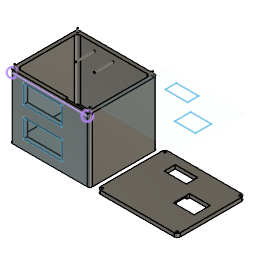
Project housingV4 (Autodesk Fusion 360 design; units mm, degrees)
Autodesk Fusion 360 part; units mm, degrees
sketch "Sketch1" plane through (0, 0, 0) normal (0, 0, 1) x (1, 0, 0)
  line L0 (2, 0) -> (63, 0)
  line L1 (65, 2) -> (65, 53)
  line L2 (63, 55) -> (2, 55)
  line L3 (0, 53) -> (0, 2)
  arc A0 (2, 55) -> (0, 53) centre (2, 53) ccw
  arc A1 (63, 0) -> (65, 2) centre (63, 2) ccw
  arc A2 (65, 53) -> (63, 55) centre (63, 53) ccw
  arc A3 (0, 2) -> (2, 0) centre (2, 2) ccw
  point P0 (65, 0)
  point P1 (0, 55)
  dimension "d1" = 55
  dimension "d2" = 65
  dimension "d3" = 2
  constraint horizontal L0
  constraint vertical L1
  constraint horizontal L2
  constraint vertical L3
  constraint coincident P1 L2
  constraint coincident P1 L3
  constraint tangent L2 A0
  constraint tangent L3 A0
  constraint coincident P0 L0
  constraint coincident P0 L1
  constraint tangent L0 A1
  constraint tangent L1 A1
  constraint equal A0 A1
  constraint tangent L1 A2
  constraint tangent L2 A2
  constraint equal A0 A2
  constraint coincident origin L0
  constraint coincident origin L3
  constraint tangent L0 A3
  constraint tangent L3 A3
  constraint equal A0 A3
  measures "d1" distance of origin P1
  measures "d2" distance of origin P0
  measures "d3" radius of A0
extrude "Extrude1" add sketch "Sketch1" along normal blind 50 makes body 1
sketch "Sketch2" plane through (0, 0, 50) normal (0, 0, 1) x (-1, 0, 0)
  arc A0 (0, -2) -> (-2, 0) centre (-2, -2) ccw
  line L0 (-2, 0) -> (-63, 0)
  arc A1 (-63, 0) -> (-65, -2) centre (-63, -2) ccw
  line L1 (-65, -2) -> (-65, -53)
  arc A2 (-65, -53) -> (-63, -55) centre (-63, -53) ccw
  line L2 (-63, -55) -> (-2, -55)
  arc A3 (-2, -55) -> (0, -53) centre (-2, -53) ccw
  line L3 (0, -53) -> (0, -2)
  line L4 (-3, -49.5) -> (-3, -5.5)
  line L5 (-5.5, -3) -> (-59.5, -3)
  line L6 (-62, -5.5) -> (-62, -49.5)
  line L7 (-59.5, -52) -> (-5.5, -52)
  arc A4 (-5.5, -52) -> (-3, -49.5) centre (-5.5, -49.5) ccw
  arc A5 (-3, -5.5) -> (-5.5, -3) centre (-5.5, -5.5) ccw
  arc A6 (-59.5, -3) -> (-62, -5.5) centre (-59.5, -5.5) ccw
  arc A7 (-62, -49.5) -> (-59.5, -52) centre (-59.5, -49.5) ccw
  dimension "d7" = 2.5
  constraint tangent L4 A4
  constraint tangent L7 A4
  constraint tangent L4 A5
  constraint tangent L5 A5
  constraint equal A4 A5
  constraint tangent L5 A6
  constraint tangent L6 A6
  constraint equal A4 A6
  constraint tangent L6 A7
  constraint tangent L7 A7
  constraint equal A4 A7
  measures "d7" radius of A4
extrude "Extrude2" cut sketch "Sketch2" against normal blind 47 contours L4 L5 L6 L7 A4 A5 A6 A7 bodies 1
sketch "Sketch3" plane through (0, 0, 0) normal (0, -1, 0) x (1, 0, 0)
  line L0 (2, 0) -> (63, 0)
  line L1 (63, 0) -> (63, 50)
  line L2 (63, 50) -> (2, 50)
  line L3 (2, 50) -> (2, 0)
sketch "Sketch4" plane through (0, 0, 0) normal (0, -1, 0) x (1, 0, 0)
  line L0 (11.3476, 47.3) -> (42.3476, 47.3)
  line L1 (42.3476, 47.3) -> (42.3476, 32.3)
  line L2 (42.3476, 32.3) -> (11.3476, 32.3)
  line L3 (11.3476, 32.3) -> (11.3476, 47.3)
  line L4 (11.3476, 23.1) -> (42.3476, 23.1)
  line L5 (11.3476, 8.1) -> (11.3476, 23.1)
  line L6 (42.3476, 8.1) -> (11.3476, 8.1)
  line L7 (42.3476, 23.1) -> (42.3476, 8.1)
  line L8 (63, 50) -> (2, 50)
  dimension "d10" = 31
  dimension "d11" = 15
  dimension "d12" = 31
  dimension "d13" = 15
  dimension "d14" = 9.2
  constraint horizontal L0
  constraint vertical L1
  constraint horizontal L2
  constraint vertical L3
  constraint horizontal L4
  constraint vertical L7
  constraint horizontal L6
  constraint vertical L5
  constraint vertical L2.end L4.start
  measures "d10" distance of L0.start L0.end
  measures "d11" distance of L0.end L1.end
  measures "d12" distance of L4.end L4.start
  measures "d13" distance of L4.end L6.start
  measures "d14" distance of L2 L4
extrude "Extrude3" cut sketch "Sketch4" against normal blind 6 bodies 1
sketch "Sketch5" plane through (0, 52, 0) normal (0, -1, 0) x (1, 0, 0)
  line L0 (59.5, 50) -> (5.5, 50)
  line L1 (5.5, 50) -> (5.5, 3)
  line L2 (5.5, 3) -> (59.5, 3)
  line L3 (59.5, 3) -> (59.5, 50)
  line L4 (15, 48) -> (33.5, 48)
  line L5 (33.5, 48) -> (33.5, 4)
  line L6 (33.5, 4) -> (15, 4)
  line L7 (15, 4) -> (15, 48)
  circle A0 centre (16.689, 46.5) radius 0.7
  circle A1 centre (31.811, 46.5) radius 0.7
  circle A2 centre (16.689, 5.5) radius 0.7
  circle A3 centre (31.811, 5.5) radius 0.7
  dimension "d18" = 44
  dimension "d19" = 18.5
  dimension "d20" = 1.4
  constraint horizontal L4
  constraint vertical L5
  constraint horizontal L6
  constraint vertical L7
  measures "d18" distance of L4.end L5.end
  measures "d19" distance of L4.start L4.end
  measures "d20" diameter of A0
extrude "Extrude4" add sketch "Sketch5" along normal blind 12 contours A0 | A1 | A2 | A3 bodies 1
sketch "Sketch6" plane through (0, 0, 50) normal (0, 0, 1) x (-1, 0, 0)
  line L0 (-5.5, -52) -> (-59.5, -52)
  arc A0 (-62, -49.5) -> (-59.5, -52) centre (-59.5, -49.5) ccw
  line L1 (-62, -49.5) -> (-62, -5.5)
  arc A1 (-59.5, -3) -> (-62, -5.5) centre (-59.5, -5.5) ccw
  line L2 (-59.5, -3) -> (-5.5, -3)
  arc A2 (-3, -5.5) -> (-5.5, -3) centre (-5.5, -5.5) ccw
  line L3 (-3, -5.5) -> (-3, -49.5)
  arc A3 (-5.5, -52) -> (-3, -49.5) centre (-5.5, -49.5) ccw
  arc A4 (0, -2) -> (-2, 0) centre (-2, -2) ccw
  line L4 (-2, 0) -> (-63, 0)
  arc A5 (-63, 0) -> (-65, -2) centre (-63, -2) ccw
  line L5 (-65, -2) -> (-65, -53)
  arc A6 (-65, -53) -> (-63, -55) centre (-63, -53) ccw
  line L6 (-63, -55) -> (-2, -55)
  arc A7 (-2, -55) -> (0, -53) centre (-2, -53) ccw
  line L7 (0, -53) -> (0, -2)
  line L8 (-2.5, -55) -> (-62.5, -55)
  line L9 (-65, -52.5) -> (-65, -2.5)
  line L10 (-62.5, 0) -> (-2.5, 0)
  line L11 (0, -2.5) -> (0, -52.5)
  arc A8 (-2.5, -55) -> (0, -52.5) centre (-2.5, -52.5) ccw
  arc A9 (-65, -52.5) -> (-62.5, -55) centre (-62.5, -52.5) ccw
  arc A10 (-62.5, 0) -> (-65, -2.5) centre (-62.5, -2.5) ccw
  arc A11 (0, -2.5) -> (-2.5, 0) centre (-2.5, -2.5) ccw
  dimension "d27" = 2.5
  constraint horizontal L8
  constraint vertical L9
  constraint horizontal L10
  constraint vertical L11
  constraint tangent L8 A8
  constraint tangent L11 A8
  constraint tangent L8 A9
  constraint tangent L9 A9
  constraint equal A8 A9
  constraint tangent L9 A10
  constraint tangent L10 A10
  constraint equal A8 A10
  constraint tangent L10 A11
  constraint tangent L11 A11
  constraint equal A8 A11
  measures "d27" radius of A8
extrude "Extrude5" add sketch "Sketch6" along normal blind 3 from surface at 1 separate body contours L0 A0 L1 A1 L2 A2 L3 A3 | L4 L5 L6 L7 L8 L9 L10 L11 A8 A9 A10 A11 makes body 2
sketch "Sketch7" plane through (0, 0, 50) normal (0, 0, 1) x (-1, 0, 0)
  line L0 (-5.5, -52) -> (-59.5, -52)
  arc A0 (-62, -49.5) -> (-59.5, -52) centre (-59.5, -49.5) ccw
  line L1 (-62, -49.5) -> (-62, -5.5)
  arc A1 (-59.5, -3) -> (-62, -5.5) centre (-59.5, -5.5) ccw
  line L2 (-59.5, -3) -> (-5.5, -3)
  arc A2 (-3, -5.5) -> (-5.5, -3) centre (-5.5, -5.5) ccw
  line L3 (-3, -5.5) -> (-3, -49.5)
  arc A3 (-5.5, -52) -> (-3, -49.5) centre (-5.5, -49.5) ccw
  arc A4 (0, -2) -> (-2, 0) centre (-2, -2) ccw
  line L4 (-2, 0) -> (-63, 0)
  arc A5 (-63, 0) -> (-65, -2) centre (-63, -2) ccw
  line L5 (-65, -2) -> (-65, -53)
  arc A6 (-65, -53) -> (-63, -55) centre (-63, -53) ccw
  line L6 (-63, -55) -> (-2, -55)
  arc A7 (-2, -55) -> (0, -53) centre (-2, -53) ccw
  line L7 (0, -53) -> (0, -2)
  circle A8 centre (-2, -53) radius 0.8549
  line L8 (-32.5, -55) -> (-32.5, 0)
  line L9 (-65, -27.5) -> (0, -27.5)
  circle A9 centre (-63, -53) radius 0.8549
  circle A10 centre (-2, -2) radius 0.8549
  circle A11 centre (-63, -2) radius 0.8549
  constraint concentric A7 A8
  constraint midpoint L6 L8.start
  constraint midpoint L4 L8.end
  constraint midpoint L5 L9.start
  constraint midpoint L7 L9.end
  constraint symmetric A8 L8 A9
  constraint symmetric A8 L9 A10
  constraint symmetric L9 A9 A11
extrude "Extrude6" cut sketch "Sketch7" along normal blind 6 contours A8 | A9 | A10 | A11 bodies 2
sketch "Sketch8" plane through (0, 0, 0) normal (0, 0, 1) x (1, 0, 0)
  circle A0 centre (2, 53) radius 0.7
  circle A1 centre (63, 53) radius 0.7
  circle A2 centre (63, 2) radius 0.7
  circle A3 centre (2, 2) radius 0.7
  dimension "d33" = 1.4
  dimension "d34" = 1.4
  dimension "d35" = 1.4
  dimension "d36" = 1.4
  measures "d33" diameter of A0
  measures "d34" diameter of A1
  measures "d35" diameter of A2
  measures "d36" diameter of A3
extrude "Extrude7" add sketch "Sketch8" along normal blind 55 bodies 1
move_body "Move1" bodies 2 to x (1, 0, 0) y (0, 1, 0) z (0, 0, 1) at (72, 0, 7)
sketch "Sketch9" plane through (0, 0, 61) normal (0, 0, 1) x (-1, 0, 0)
  circle A0 centre (-135, -53) radius 0.8549
  circle A1 centre (-135, -2) radius 0.8549
  circle A2 centre (-74, -53) radius 0.8549
  circle A3 centre (-74, -2) radius 0.8549
  arc A4 (-74.5, -55) -> (-72, -52.5) centre (-74.5, -52.5) ccw
  line L0 (-72, -52.5) -> (-72, -2.5)
  arc A5 (-72, -2.5) -> (-74.5, 0) centre (-74.5, -2.5) ccw
  line L1 (-74.5, 0) -> (-134.5, 0)
  arc A6 (-134.5, 0) -> (-137, -2.5) centre (-134.5, -2.5) ccw
  line L2 (-137, -2.5) -> (-137, -52.5)
  arc A7 (-137, -52.5) -> (-134.5, -55) centre (-134.5, -52.5) ccw
  line L3 (-134.5, -55) -> (-74.5, -55)
  line L4 (-130, -33.8) -> (-113.25, -33.8)
  line L5 (-113.25, -33.8) -> (-113.25, -20.8)
  line L6 (-113.25, -20.8) -> (-130, -20.8)
  line L7 (-130, -20.8) -> (-130, -33.8)
  line L8 (-87.0382, -48.325) -> (-105.1641, -48.325)
  line L9 (-105.1641, -48.325) -> (-105.1641, -39.325)
  line L10 (-105.1641, -39.325) -> (-87.0382, -39.325)
  line L11 (-87.0382, -39.325) -> (-87.0382, -48.325)
  dimension "d39" = 16.75
  dimension "d40" = 13
  dimension "d43" = 9
  constraint horizontal L4
  constraint vertical L5
  constraint horizontal L6
  constraint vertical L7
  constraint horizontal L8
  constraint vertical L9
  constraint horizontal L10
  constraint vertical L11
  measures "d39" distance of L4.start L4.end
  measures "d40" distance of L4.start L6.end
  measures "d43" distance of L8.start L10.end
extrude "Extrude8" cut sketch "Sketch9" against normal blind 13 contours L4 L5 L6 L7 bodies 2
extrude "Extrude9" cut sketch "Sketch9" against normal blind 16 contours L8 L9 L10 L11 bodies 2
move_body "Move2" bodies 2 to x (1, 0, 0) y (0, 1, 0) z (0, 0, 1) at (-71.997, 0.0813, 0)
move_body "Move3" bodies 2 to x (1, 0, 0) y (0, 1, 0) z (0, 0, 1) at (71, 0, -58)
extrude "Extrude10" add 1 faces at (23.5, 1, 50) along direction (0, 0, 1) blind 2 on bodies 1 bodies 1
sketch "Sketch11" plane through (0, 0, 52) normal (0, 0, 1) x (-1, 0, 0)
  circle A0 centre (-2, -2) radius 0.7
  circle A1 centre (-2, -53) radius 0.7
  circle A2 centre (-63, -2) radius 0.7
  circle A3 centre (-63, -53) radius 0.7
  line L0 (-5.5, -52) -> (-59.5, -52)
  arc A4 (-62, -49.5) -> (-59.5, -52) centre (-59.5, -49.5) ccw
  line L1 (-62, -49.5) -> (-62, -5.5)
  arc A5 (-59.5, -3) -> (-62, -5.5) centre (-59.5, -5.5) ccw
  line L2 (-59.5, -3) -> (-5.5, -3)
  arc A6 (-3, -5.5) -> (-5.5, -3) centre (-5.5, -5.5) ccw
  line L3 (-3, -5.5) -> (-3, -49.5)
  arc A7 (-5.5, -52) -> (-3, -49.5) centre (-5.5, -49.5) ccw
  arc A8 (0, -2) -> (-2, 0) centre (-2, -2) ccw
  line L4 (-2, 0) -> (-63, 0)
  arc A9 (-63, 0) -> (-65, -2) centre (-63, -2) ccw
  line L5 (-65, -2) -> (-65, -53)
  arc A10 (-65, -53) -> (-63, -55) centre (-63, -53) ccw
  line L6 (-63, -55) -> (-2, -55)
  arc A11 (-2, -55) -> (0, -53) centre (-2, -53) ccw
  line L7 (0, -53) -> (0, -2)
  line L8 (-44, -3) -> (-58, -3)
  line L9 (-58, -3) -> (-58, -1.5)
  line L10 (-58, -1.5) -> (-44, -1.5)
  line L11 (-44, -1.5) -> (-44, -3)
  constraint horizontal L8
  constraint vertical L9
  constraint horizontal L10
  constraint vertical L11
  constraint coincident L2 L8.start
extrude "Extrude11" cut sketch "Sketch11" against normal blind 47 contours L2 L8 L9 L10 L11 bodies 1
extrude "Extrude12" add 4 faces at (16.7409, 40, 46.2725) (31.4478, 40, 46.6314) (31.6656, 40, 5.6824) (16.4731, 40, 5.7327) along direction (0, -1, 0) blind 3 on bodies 1 bodies 1
sketch "Sketch12" plane through (0, 0, 0) normal (0, 0, -1) x (1, 0, 0)
  line L0 (104.1671, -39.4063) -> (104.1671, -48.4063)
  line L1 (104.1671, -48.4063) -> (86.0412, -48.4063)
  line L2 (86.0412, -48.4063) -> (86.0412, -39.4063)
  line L3 (86.0412, -39.4063) -> (104.1671, -39.4063)
  line L4 (129.003, -33.8813) -> (112.253, -33.8813)
  line L5 (112.253, -33.8813) -> (112.253, -20.8813)
  line L6 (112.253, -20.8813) -> (129.003, -20.8813)
  line L7 (129.003, -20.8813) -> (129.003, -33.8813)
  circle A0 centre (134.003, -53.0813) radius 0.8549
  circle A1 centre (134.003, -2.0813) radius 0.8549
  circle A2 centre (73.003, -53.0813) radius 0.8549
  circle A3 centre (73.003, -2.0813) radius 0.8549
  arc A4 (71.003, -52.5813) -> (73.503, -55.0813) centre (73.503, -52.5813) ccw
  line L8 (73.503, -55.0813) -> (133.503, -55.0813)
  arc A5 (133.503, -55.0813) -> (136.003, -52.5813) centre (133.503, -52.5813) ccw
  line L9 (136.003, -52.5813) -> (136.003, -2.5813)
  arc A6 (136.003, -2.5813) -> (133.503, -0.0813) centre (133.503, -2.5813) ccw
  line L10 (133.503, -0.0813) -> (73.503, -0.0813)
  arc A7 (73.503, -0.0813) -> (71.003, -2.5813) centre (73.503, -2.5813) ccw
  line L11 (71.003, -2.5813) -> (71.003, -52.5813)
  line L12 (87, -27.3813) -> (87, -23)
  line L13 (87, -23) -> (112.253, -23)
  line L14 (87, -31.7625) -> (112.253, -31.7625)
  line L15 (87, -27.3813) -> (87, -31.7625)
  constraint coincident L5 L13.end
  constraint perpendicular L5 L13
extrude "Extrude13" cut sketch "Sketch12" against normal blind 2 contours L5 L12 L13 L14 L15 bodies 2
